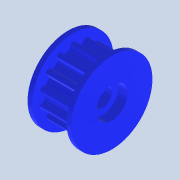
# Autodesk Inventor part: HTPT14S5M100-A-H6_b
Saved by Autodesk Inventor 2021.2 (Build 252289000, 289)
## iProperties
Category: PARTsolutions
Company: MISUMI
Part Number: HTPT14S5M100-A-H6_b
Material: ABS プラスチック
Catalog Web Link: www.cadenas.de
Description: HTPA__S5M100, HTPA__S5M150, HTPA__S5M250, HTPB__S5M100, HTPB__S5M150, HTPB__S5M250, HTPK__S5M100, HTPK__S5M150, HTPK__S5M250, HTPN__S5M100, HTPN__S5M150, HTPN__S5M250, HTPT__S5M100, HTPT__S5M150, HTPT__S5M250, HTPM__S5M100, HTPM__S5M150, HTPM__S5M250, HTPP__S5M100, HTPP__S5M150, HTPP__S5M250, HTPS__S5M100, HTPS__S5M150_body-High Torque Timing Pulleys S5M Type
Vendor: MISUMI
Document SubType Name: Modeling
Designer: partserver
Manufacturer: MISUMI
Mass: 4.76405 g
Surface Area: 30.9583 cm^2
Volume: 4.76405 cm^3
Density: 1.06 g/cm^3
Appearance: 青 - 壁塗料 - 光沢
PSOL_IDENT_0: {$CADENAS_DATA\23d-libs\misumi\metric\51_timing_pulleys\htpb_s5m\htpb_s5m.prj},732 {VTYP=3D},{NB=HTP
PSOL_IDENT_1: T14S5M100-A-H6_b},{LINA=HTPT14S5M100-A-H6},{NN=HTPA__S5M100, HTPA__S5M150, HTPA__S5M250, HTPB__S5M10
PSOL_IDENT_2: 0, HTPB__S5M150, HTPB__S5M250, HTPK__S5M100, HTPK__S5M150, HTPK__S5M250, HTPN__S5M100, HTPN__S5M150,
PSOL_IDENT_3: HTPN__S5M250, HTPT__S5M100, HTPT__S5M150, HTPT__S5M250, HTPM__S5M100, HTPM__S5M150, HTPM__S5M250, H
PSOL_IDENT_4: TPP__S5M100, HTPP__S5M150, HTPP__S5M250, HTPS__S5M100, HTPS__S5M150_body},{DATE=17.01.2019 01:25:31}
PSOL_IDENT_5: ,{GEOMDATE=28.12.2018 04:09:27},{VERSION=},{LINEID=10},{WBVAR=MATP,ST,TNW,PS,SBS,DD,Z,J,Q,R,S,T,ALT1
PSOL_IDENT_6: ,ALT2,M,QSC,QFC,QTC,ALT3,K,KSC,KFC,KTC,ALT4,ZM,ZSC,ZFC,ZTC,ALT5,ALT6,ALT7,FC,ALT8,SRG,ALT9,BTC,TL,AL
PSOL_IDENT_7: T10,TPC,ALT11,BC,ALT12,SLH},{WBNUMERIC=DD,Z,J,Q,R,S,T,QSC,QFC,QTC,K,KSC,KFC,KTC,ZSC,ZFC,ZTC,FC,SRG,B
PSOL_IDENT_8: TC,TL,BC,SLH}  {NB=HTPT14S5M100-A-H6_b},{LINA=HTPT14S5M100-A-H6},{KT=DUMMY},{PN=HTPT14S5M100-A-H6},{
PSOL_IDENT_9: TYPE=HTPT},{MATP=S45C},{MATPALG= 'A2017','Aluminum Alloy 2000 series','S45C','1045 Carbon Steel Equi
PSOL_IDENT_10: valent','SUS304','SUS304' },{ST=-},{STALG= '-','-','BO','Black Oxide','ENP','Electroless Nickel Plat
PSOL_IDENT_11: ing' },{NT=14},{TNW=S5M100},{TNWALG= 'S5M100','S5M150','S5M250' },{BW=10},{PS=A},{PSALG= 'A','B' },{
PSOL_IDENT_12: SBS=H},{SBSALG= 'H','Round Hole','P','Round Hole + Tap','N','New JIS Keywayed Bore + Tap (Standard)'
PSOL_IDENT_13: ,'NK','New JIS Keywayed Bore + Tap (width 4.0mm, height 1.8mm)','C','Old JIS Keywayed Bore + Tap','V'
PSOL_IDENT_14: ,'Stepped Hole','Y','Both Ends Stepped Hole','WB','Double Stepped Hole' },{DD=6.00},{DDALG=[5:6/1],6
PSOL_IDENT_15: .35,[7:12/1]},{DDHA=[5:6/1],6.35,[7:12/1]},{DDPA=[5:6/1],6.35,[7:10/1]},{DDNA=[8:8/1],[10:10/1]},{DD
PSOL_IDENT_16: CA=[10]},{DDVA=[5:6/1],6.35,[7:10/1]},{DDY=[5:10/1]},{DDWB=[5:8/1]},{DDHB=},{DDPB=},{DDNB=},{DDNK=[1
PSOL_IDENT_17: 0:10/1]},{DDCB=},{DDVFB=},{Z=0},{ZALG=[0]},{ZMIN=8.000},{ZAMAX=12.000},{ZBMAX=0.000},{DDZ=6.000},{J=
PSOL_IDENT_18: 0.0},{JALG=[0]},{JMIN=2.000},{JMAX=14.000},{JPN=},{Q=0},{QALG=[0]},{QRMIN=8.000},{QRMAX=12.000},{WBQ
PSOL_IDENT_19: MIN=10.000},{R=0},{RALG=[0]},{WBRMAX=-2.000},{S=0.0},{SALG=[0]},{SMAX=10.000},{T=0.0},{TALG=[0]},{TM
PSOL_IDENT_20: AX=13.000},{SBSPN=-H6},{A=11},{W=16},{L=0},{PD=22.28},{OD=21.32},{D=0},{DALG=14.000},{DE=16.000},{F=
PSOL_IDENT_21: 26},{E=16},{TT=1.6},{BBK=0.000},{TTK=0.000},{ALT1=},{ALT1ALG= '','Not applicable' },{ANG=128.571},{A
PSOL_IDENT_22: LT1PN=},{ALT2=},{ALT2ALG= '','Not applicable' },{M=N/A},{MALG= 'N/A' },{MFTALG= 'N/A' },{MSALG= 'N/A'
PSOL_IDENT_23: },{M3D=0.000},{KDML=0.000},{ML=0.000},{MUL=0.000},{PITCH=0.000},{QSC=0.0},{QSCALG=0},{QFC=0.0},{QFC
PSOL_IDENT_24: ALG=0},{QTC=0.0},{QTCALG=0},{QPCDMIN=0.000},{QPCDMINALG=0.000},{QPCDMAX=12.000},{ALT2PN=},{TAP=0.000
PSOL_IDENT_25: },{ALT3=},{ALT3ALG= '','Not applicable' },{K=0.0},{KALG=0},{KMIN=4.000},{KFTMAX=0.000},{KSMAX=0.000}
PSOL_IDENT_26: ,{KSC=0.0},{KSCALG=0},{KFC=0.0},{KFCALG=0},{KTC=0.0},{KTCALG=0},{KSCMIN=10.000},{KSCMINALG=10},{KPCD
PSOL_IDENT_27: MIN=10.000},{KPCDMINALG=10},{KPCDMAX=12.000},{ALT3PN=},{ALT4=},{ALT4ALG= '','Not applicable' },{ALT4
PSOL_IDENT_28: MIN=16.500},{ALT4MAX=5.500},{ZM=N/A},{ZMALG= 'N/A' },{ZMFTALG= 'N/A' },{ZMSALG= 'N/A' },{ZMDD1=0.0},
PSOL_IDENT_29: {ZMDD2=0.0},{ZMHH=0.0},{ZSC=0.0},{ZSCALG=[0]},{ZFC=0.0},{ZFCALG=[0]},{ZTC=0.0},{ZTCALG=[0]},{ZPCDMIN=
PSOL_IDENT_30: 0.000},{ZPCDMINALG=0.000},{ZPCDMAX=12.000},{ALT4PN=},{ALT5=},{ALT5ALG= '','w/o Flange not Attached','
PSOL_IDENT_31: NFC','with NFC (Flange not Attached)' },{ALT5PN=},{ALT6=},{ALT6ALG= '','w/o Flange Attached on One S
PSOL_IDENT_32: ide Only','RFC','with RFC (Flange Attached on The Boss Side Only)','LFC','with LFC (Flange Attached
PSOL_IDENT_33: on The Opposite Side Only)' },{ALT6PN=},{ALT7=},{ALT7ALG= '','w/o FC (Flange Cut)','FC','with FC (Fl
PSOL_IDENT_34: ange Cut)' },{FC=0.0},{FCALG=0},{FCMIN=22.5},{FCMAX=24.0},{ALT7PN=},{ALT8=},{ALT8ALG= '','Not applic
PSOL_IDENT_35: able' },{ALT8ALGALG=12.000},{ALT8DD2=0.000},{ALT8MM=0.000},{ALT8NN=0.000},{QC=0.000},{KC=0.000},{ZC=
PSOL_IDENT_36: 0.000},{SRG=0.0},{SRGALG=[0]},{SRGMAX=0.000},{DD2=0.0},{MM=0.00},{NN=0.00},{ALT8PN=},{ALT9=},{ALT9AL
PSOL_IDENT_37: G= '','w/o BTC (Taper for Bearing Holder)','BTC','with BTC (Taper for Bearing Holder)' },{BTC9=8.000
PSOL_IDENT_38: },{TL9=1.000},{BTC=0},{BTCALG=[0]},{TL=0.0},{TLALG=0},{TLMIN=1.000},{TLMAX=-16.500},{BTCL=0},{BTCD=0
PSOL_IDENT_39: },{ALT9PN=},{WLBCTL=16.000},{ALT10=},{ALT10ALG= '','Not applicable' },{TPC=N/A},{TPCALG= 'N/A' },{TP
PSOL_IDENT_40: CM=4.000},{ALT10PN=},{ALT11=},{ALT11ALG= '','Not applicable' },{BC=0.0},{BCALG=0},{BCMIN=3.000},{BCM
PSOL_IDENT_41: AX=-16.500},{M1WBC=8.000},{ALT11PN=},{KTT=7.660},{ALT12=},{ALT12ALG= '','Not applicable' },{SLH=0},{
PSOL_IDENT_42: SLHALG=[0]},{ALT12PN=},{AC=-},{M1=4.000},{M1L=3.000}
NB: HTPT14S5M100-A-H6_b
NN: 0
NT: 14
NBSYN: $PN._b
LINA: HTPT14S5M100-A-H6
CATALOG: Misumi
PN: HTPT14S5M100-A-H6
MATP: 1045 Carbon Steel Equivalent
ST: -
TNW: S5M100
BW: 10
PS: A
SBS: Round Hole
DD: 6
Z: 0
J: 0
Q: 0
R: 0
S: 0
T: 0
A: 11
W: 16
L: 0
PD: 22.28
OD: 21.32
D: 0
F: 26
E: 16
TT: 1.6
ALT1: Not applicable
ALT2: Not applicable
M: N/A
QSC: 0
QFC: 0
QTC: 0
ALT3: Not applicable
K: 0
KSC: 0
KFC: 0
KTC: 0
ALT4: Not applicable
ZM: N/A
ZMDD1: 0
ZMDD2: 0
ZMHH: 0
ZSC: 0
ZFC: 0
ZTC: 0
ALT5: w/o Flange not Attached
ALT6: w/o Flange Attached on One Side Only
ALT7: w/o FC (Flange Cut)
FC: 0
ALT8: Not applicable
SRG: 0
DD2: 0
MM: 0
ALT9: w/o BTC (Taper for Bearing Holder)
BTC: 0
TL: 0
BTCL: 0
BTCD: 0
ALT10: Not applicable
TPC: N/A
ALT11: Not applicable
BC: 0
ALT12: Not applicable
SLH: 0
AC: -
SUPPLIER: MISUMI
ARTICLENO: HTPT14S5M100-A-H6_b
BOMINFO: HTPT14S5M100-A-H6
CREATOR: CADENAS GmbH
Title: HTPT14S5M100-A-H6
Author: Cadenas PARTsolutions
Comments: High Torque Timing Pulleys S5M Type
Autodesk Inventor part; units mm, degrees
note: some values were not read from the file. Chosen so that the rebuilt part matches the saved one: pattern direction of "Circular Pattern1".
ref_plane "YZ Plane" through (0, 0, 0) normal (1, 0, 0) x (0, 1, 0)
ref_plane "XZ Plane" through (0, 0, 0) normal (0, 1, 0) x (-1, 0, 0)
ref_plane "XY Plane" through (0, 0, 0) normal (0, 0, 1) x (1, 0, 0)
sketch "_____2" plane through (0, 0, 0) normal (0, 0, 1) x (1, 0, 0)
  line L0 (16, 0) -> (0, 0)
  line L1 (0, 0) -> (0, 8)
  line L2 (0, 8) -> (0.9, 8)
  line L3 (0.9, 8) -> (0.9, 10.449356)
  line L4 (0.9, 10.449356) -> (0.327518, 12.58589)
  line L5 (0.327518, 12.58589) -> (1.872999, 13)
  line L6 (1.872999, 13) -> (2.5, 10.66)
  line L7 (2.5, 10.66) -> (13.5, 10.66)
  line L8 (13.5, 10.66) -> (14.127001, 13)
  line L9 (14.127001, 13) -> (15.672482, 12.58589)
  line L10 (15.672482, 12.58589) -> (15.1, 10.449356)
  line L11 (15.1, 10.449356) -> (15.1, 8)
  line L12 (15.1, 8) -> (16, 8)
  line L13 (16, 8) -> (16, 0)
  line L14 (16, 0) -> (0, 0)
  constraints: 30 end point
revolve "Revolution1" add sketch "_____2" angle 360 about axis through (16, 0, 0) along (1, 0, 0)
sketch "Sketch2" plane through (16, 0, 0) normal (1, 0, 0) x (0, 0, -1)
  point P0 (0, 0)
hole "Hole1" at (16, 0, 0) direction (-1, 0, 0) diameter 6 depth 16
sketch "_____6" plane through (2.5, 0, 0) normal (1, 0, 0) x (0, 0, -1)
  arc A0 (-1.507142, 10.064124) -> (-2.143757, 10.442217) centre (-2.033151, 9.903454) ccw
  arc A1 (-1.507142, 10.064124) -> (-0.915185, 8.953699) centre (1.625, 11.020843) ccw
  arc A2 (-0.915185, 8.953699) -> (-0.701549, 8.862276) centre (-0.721278, 9.111496) ccw
  arc A3 (0.701549, 8.862276) -> (-0.701549, 8.862276) centre (0, 0) ccw
  arc A4 (0.701549, 8.862276) -> (0.915185, 8.953699) centre (0.721278, 9.111496) ccw
  arc A5 (0.915185, 8.953699) -> (1.507142, 10.064124) centre (-1.625, 11.020843) ccw
  arc A6 (2.143757, 10.442217) -> (1.507142, 10.064124) centre (2.033151, 9.903454) ccw
  line L0 (2.143757, 10.442217) -> (2.143757, 10.931784)
  arc A7 (2.143757, 10.931784) -> (-2.143757, 10.931784) centre (0, 0) ccw
  line L1 (-2.143757, 10.931784) -> (-2.143757, 10.442217)
  constraints: 16 point on circle, 8 centre point, 4 end point
extrude "Extrusion1" cut sketch "_____6" along normal blind 11
pattern_circular "Circular Pattern1" count 14 over 360 about axis through (2.5, 0, 0) along (1, 0, 0) of "Extrusion1"
sketch "スケッチ4" plane through (0, 0, 0) normal (-1, 0, 0) x (0, 0, 1)
  circle A0 centre (0, 0) radius 13 projected
  circle A1 centre (0, 0) radius 3 projected
extrude "押し出し2" add sketch "スケッチ4" against normal up to surface (2.5 mm away)
sketch "スケッチ5" plane through (0, 0, 0) normal (-1, 0, 0) x (0, 0, 1)
  circle A0 centre (0, 0) radius 13 projected
extrude "押し出し3" cut sketch "スケッチ5" against normal blind 1
sketch "スケッチ6" plane through (16, 0, 0) normal (1, 0, 0) x (0, 0, -1)
  circle A0 centre (0, 0) radius 13 projected
  circle A1 centre (0, 0) radius 3 projected
extrude "押し出し4" add sketch "スケッチ6" against normal up to surface (2.5 mm away)
sketch "スケッチ7" plane through (16, 0, 0) normal (1, 0, 0) x (0, 0, -1)
  circle A0 centre (0, 0) radius 13 projected
extrude "押し出し5" cut sketch "スケッチ7" against normal blind 1
sketch "スケッチ8" plane through (1, 0, 0) normal (-1, 0, 0) x (0, 0, 1)
  point P0 (0, 0)
  point P1 (0, 0)
  constraints: 1 coincident
hole "穴2" at (1, 0, 0) direction (1, 0, 0) diameter 10 depth 3
sketch "スケッチ9" plane through (15, 0, 0) normal (1, 0, 0) x (0, 0, -1)
  point P0 (0, 0)
  point P1 (0, 0)
  constraints: 1 coincident
hole "穴3" at (15, 0, 0) direction (-1, 0, 0) diameter 10 depth 3
body "Solid1"
